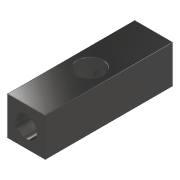
# Autodesk Inventor part: stelblokje
Saved by Autodesk Inventor 2020.3 (Build 243373000, 373)
## iProperties
Created: 2020-09-15
Part Number: stelblokje
Material: Stainless Steel
Document SubType Name: Modeling
Designer: Svend
Density: 8 g/cm^3
Appearance: Semi-Polished
Author: Svend
Autodesk Inventor part; units mm, degrees
ref_plane "YZ Plane" through (0, 0, 0) normal (1, 0, 0) x (0, 1, 0)
ref_plane "XZ Plane" through (0, 0, 0) normal (0, 1, 0) x (-1, 0, 0)
ref_plane "XY Plane" through (0, 0, 0) normal (0, 0, 1) x (1, 0, 0)
sketch "Sketch1" plane through (0, 0, 0) normal (0, 0, 1) x (1, 0, 0)
  line L0 (-7.5, 7.5) -> (7.5, 7.5)
  line L1 (7.5, 7.5) -> (7.5, -7.5)
  line L2 (7.5, -7.5) -> (-7.5, -7.5)
  line L3 (-7.5, -7.5) -> (-7.5, 7.5)
  line L4 (-7.5, 7.5) -> (7.5, -7.5) construction
  line L5 (7.5, 7.5) -> (-7.5, -7.5) construction
  circle A0 centre (0, 0) radius 4.1
  dimension "d0" = 15
  dimension "d1" = 15
  dimension "d2" = 8.2
  constraints: 12 end point, 2 midpoint, 2 parallel, 1 centre point, 1 coincident, 1 horizontal, 1 perpendicular
  measures "d0" distance of L1.end L2.end
  measures "d1" distance of L0.end L1.end
  measures "d2" diameter of A0
extrude "Extrusion1" add sketch "Sketch1" along normal mid plane 50
sketch "Sketch2" plane through (-7.5, 7.5, 25) normal (0, 1, 0) x (1, 0, 0)
  circle A0 centre (7.5, 25) radius 5.1
  dimension "d5" = 10.2
  constraints: 1 centre point, 1 coincident
  measures "d5" diameter of A0
extrude "Extrusion2" cut sketch "Sketch2" against normal through all
fillet "Fillet1" radius 0.2 18 edges at (-4.1, 0, 25) (0, -7.5, -25) (-7.5, -7.5, 0) (0, -7.5, 25) (7.5, -7.5, 0) (0, 7.5, -25) (7.5, 7.5, 0) (0, 7.5, 25) (-7.5, 7.5, 0) (-4.1, 0, -25) (-5.1, 7.5, 0) (-5.1, -7.5, 0) (-4.0999, 0.026, -3.0333) (-4.0999, 0.026, 3.0333) (7.5, 0, 25) (-7.5, 0, 25) (7.5, 0, -25) (-7.5, 0, -25)
body "Solid1"
